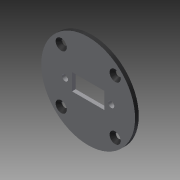
# Autodesk Inventor part: anschluss_daten
Saved by Autodesk Inventor 2015 (Build 190159000, 159)
## iProperties
Created: 2018-04-03
Part Number: anschluss_daten
Material: Generisch
Document SubType Name: Modeling
Designer: wepet
Density: 1 g/cm^3
Appearance: Vorgabe
Author: wepet
Autodesk Inventor part; units mm, degrees
ref_plane "YZ Plane" through (0, 0, 0) normal (1, 0, 0) x (0, 1, 0)
ref_plane "XZ Plane" through (0, 0, 0) normal (0, 1, 0) x (-1, 0, 0)
ref_plane "XY Plane" through (0, 0, 0) normal (0, 0, 1) x (1, 0, 0)
sketch "Skizze1" plane through (0, 0, 0) normal (0, 1, 0) x (-1, 0, 0)
  circle A0 centre (0, 0) radius 25.4
  dimension "d0" = 50.8
  constraints: 1 centre point, 1 coincident
  measures "d0" diameter of A0
extrude "Extrusion1" add sketch "Skizze1" along normal blind 2
sketch "Skizze2" plane through (0, 0, 0) normal (0, -1, 0) x (1, 0, 0)
  circle A0 centre (0, 0) radius 25.4 projected
  line L0 (-14.6, 14.6) -> (14.6, 14.6) construction
  line L1 (14.6, 14.6) -> (14.6, -14.6) construction
  line L2 (14.6, -14.6) -> (-14.6, -14.6) construction
  line L3 (-14.6, -14.6) -> (-14.6, 14.6) construction
  line L4 (0, 0) -> (14.6, 0) construction
  line L5 (0, 0) -> (0, 14.6) construction
  dimension "d3" = 29.2
  dimension "d4" = 29.2
  constraints: 12 end point, 4 coincident, 2 horizontal, 2 midpoint, 2 parallel, 1 perpendicular, 1 vertical
  measures "d3" distance of L0.start L0.end
  measures "d4" distance of L0.end L1.end
hole "Bohrung1" at (-14.6, 0, 14.6) at (14.6, 0, 14.6) at (14.6, 0, -14.6) at (-14.6, 0, -14.6) direction (0, 1, 0) diameter 3 end through all countersink diameter 6 countersink angle 90
sketch "Skizze7" plane through (0, 0, 0) normal (0, -1, 0) x (1, 0, 0)
  circle A0 centre (0, 0) radius 25.4 projected
  line L0 (-8.75, 4.5) -> (8.75, 4.5)
  line L1 (8.75, 4.5) -> (8.75, -4.5)
  line L2 (8.75, -4.5) -> (-8.75, -4.5)
  line L3 (-8.75, -4.5) -> (-8.75, 4.5)
  line L4 (0, 0) -> (8.75, 0) construction
  line L5 (0, 0) -> (0, 4.5) construction
  line L6 (0, 0) -> (12.5, 0) construction
  line L7 (0, 0) -> (-12.5, 0) construction
  dimension "d25" = 17.5
  dimension "d26" = 9
  dimension "d28" = 12.5
  dimension "d29" = 12.5
  constraints: 16 end point, 3 perpendicular, 2 coincident, 2 horizontal, 2 midpoint, 2 parallel, 1 point on line
  measures "d25" distance of L0.start L0.end
  measures "d26" distance of L2.end L0.start
  measures "d28" distance of L4.start L6.end
  measures "d29" distance of L4.start L7.end
extrude "Extrusion5" cut sketch "Skizze7" against normal blind 2 contours L0 L1 L2 L3
sketch "Skizze8" plane through (0, 0, 0) normal (0, -1, 0) x (1, 0, 0)
  circle A0 centre (0, 0) radius 25.4 projected
  line L0 (0, 0) -> (12.5, 0) construction
  line L1 (0, 0) -> (-12.5, 0) construction
  dimension "d32" = 12.5
  dimension "d33" = 12.5
  constraints: 4 end point, 2 coincident, 2 horizontal
  measures "d32" distance of L0.start L0.end
  measures "d33" distance of L0.start L1.end
hole "Bohrung2" at (-12.5, 0, 0) at (12.5, 0, 0) direction (0, 1, 0) diameter 3.3 end through all
